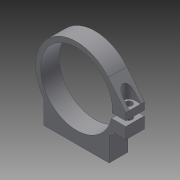
# Autodesk Inventor part: Motor Mount
Saved by Autodesk Inventor 2014 SP1 (Build 180222100, 222)
## iProperties
Created: 2014-01-12
Part Number: Motor Mount
Material: Generic
Document SubType Name: Modeling
Designer: tom
Density: 1 g/cm^3
Appearance: Default
Author: tom
Autodesk Inventor part; units mm, degrees
ref_plane "YZ Plane" through (0, 0, 0) normal (1, 0, 0) x (0, 1, 0)
ref_plane "XZ Plane" through (0, 0, 0) normal (0, 1, 0) x (-1, 0, 0)
ref_plane "XY Plane" through (0, 0, 0) normal (0, 0, 1) x (1, 0, 0)
sketch "Sketch1" plane through (0, 0, 0) normal (0, 0, 1) x (1, 0, 0)
  arc A0 (18.3475, -1.5748) -> (17.9494, -4.1148) centre (0, 0) ccw
  line L0 (-16.7386, -24.5618) -> (16.7386, -24.5618)
  line L1 (16.7386, -24.5618) -> (16.7386, -12.6068)
  line L2 (-16.7386, -12.6068) -> (-16.7386, -24.5618)
  line L3 (-20.955, 0) -> (-20.955, 20.955) construction
  line L4 (-20.955, 20.955) -> (25.273, 20.955) construction
  line L5 (16.7386, -24.5618) -> (25.273, -24.5618) construction
  line L6 (25.273, -24.5618) -> (25.273, -9.9568) construction
  line L7 (25.273, -9.9568) -> (21.0058, -9.9568) construction
  line L8 (25.273, -9.9568) -> (25.273, 2.1082) construction
  line L9 (25.273, 2.1082) -> (16.2735, 13.2017)
  line L10 (25.273, 2.1082) -> (25.273, -1.5748) construction
  line L11 (25.273, -1.5748) -> (18.3475, -1.5748)
  line L12 (25.273, 2.1082) -> (25.273, -1.5748)
  line L13 (25.273, -1.5748) -> (25.273, -4.1148) construction
  line L14 (25.273, -4.1148) -> (25.273, -9.9568)
  line L15 (25.273, -9.9568) -> (18.4384, -9.9568)
  line L16 (25.273, -4.1148) -> (17.9494, -4.1148)
  arc A1 (16.2735, 13.2017) -> (-16.7386, -12.6068) centre (0, 0) ccw
  arc A2 (16.7386, -12.6068) -> (18.4384, -9.9568) centre (0, 0) ccw
  dimension "d0" = 36.83
  constraints: 34 end point, 7 perpendicular, 7 point on circle, 3 centre point, 3 parallel, 2 coincident, 2 point on line, 2 tangent, 1 collinear
  measures "d0" diameter of A0
extrude "Extrusion1" add sketch "Sketch1" along normal blind 9.525
sketch "Sketch2" plane through (-16.7386, -24.5618, 0) normal (0, -1, 0) x (1, 0, 0)
  line L0 (0, 9.525) -> (33.4772, 9.525) projected
  line L1 (16.7386, 0) -> (16.7386, 9.525) construction
  line L2 (30.2133, 4.7625) -> (3.2639, 4.7625) construction
  circle A0 centre (3.2639, 4.7625) radius 1.7526
  circle A1 centre (30.2133, 4.7625) radius 1.7526
  dimension "d12" = 26.9494
  dimension "d13" = 3.5052
  dimension "d14" = 3.5052
  constraints: 4 end point, 2 centre point, 2 coincident, 1 midpoint
  measures "d12" distance of L2.start L2.end
  measures "d13" diameter of A0
  measures "d14" diameter of A1
extrude "Extrusion2" cut sketch "Sketch2" against normal blind 9.525
thread "Thread1" size "6-32 UNC" class "2B" standard "ANSI Unified Screw Threads" full length
thread "Thread2" size "6-32 UNC" class "2B" standard "ANSI Unified Screw Threads" full length
sketch "Sketch3" plane through (18.4384, -9.9568, 0) normal (0, -1, 0) x (1, 0, 0)
  line L0 (6.8346, 0) -> (6.8346, 9.525) projected
  line L1 (0, 0) -> (0, 9.525) projected
  line L2 (6.8346, 4.7625) -> (3.6596, 4.7625) construction
  circle A0 centre (3.6596, 4.7625) radius 1.7526
  point P0 (-18.4384, 0)
  dimension "d21" = 3.175
  dimension "d22" = 3.5052
  constraints: 2 end point, 1 centre point, 1 coincident, 1 midpoint, 1 perpendicular
  measures "d21" distance of L2.start L2.end
  measures "d22" diameter of A0
extrude "Extrusion3" cut sketch "Sketch3" against normal blind 25.4
sketch "Sketch4" plane through (25.273, -1.5748, 0) normal (1, 0, 0) x (0, 0, -1)
  line L0 (0, 3.683) -> (-9.525, 3.683) projected
  line L1 (-1.8415, 3.683) -> (-7.6835, 3.683)
  line L2 (-7.6835, 3.683) -> (-7.6835, 13.843)
  line L3 (-7.6835, 13.843) -> (-1.8415, 13.843)
  line L4 (-1.8415, 13.843) -> (-1.8415, 3.683)
  point P0 (0, 1.5748)
  dimension "d26" = 10.16
  dimension "d27" = 5.842
  constraints: 8 end point, 2 perpendicular, 2 point on line, 1 parallel
  measures "d26" distance of L1.end L2.end
  measures "d27" distance of L2.end L3.end
extrude "Extrusion4" cut sketch "Sketch4" against normal blind 3.175
sketch "Sketch5" plane through (25.273, 2.1082, 7.6835) normal (0, 1, 0) x (1, 0, 0)
  arc A0 (-3.175, 1.1684) -> (-3.175, 4.6736) centre (-3.175, 2.921) ccw projected
  circle A1 centre (-3.175, 2.921) radius 2.921
  point P0 (-25.273, 7.6835)
  constraints: 1 centre point, 1 coincident
extrude "Extrusion5" cut sketch "Sketch5" along normal blind 9.525
thread "Thread3" size "6-32 UNC" class "2B" standard "ANSI Unified Screw Threads" full length
body "Solid1"
